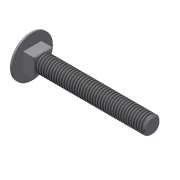
# Autodesk Inventor part: Šroub M10x70
Saved by Autodesk Inventor 2015 (Build 190159000, 159)
## iProperties
Created: 2015-07-31
Part Number: Šroub M10x70
Material: Všeobecné
Document SubType Name: Modeling
Designer: Michal
Density: 1 g/cm^3
Appearance: Výchozí
Author: Michal
Autodesk Inventor part; units mm, degrees
ref_plane "YZ Plane" through (0, 0, 0) normal (1, 0, 0) x (0, 1, 0)
ref_plane "XZ Plane" through (0, 0, 0) normal (0, 1, 0) x (-1, 0, 0)
ref_plane "XY Plane" through (0, 0, 0) normal (0, 0, 1) x (1, 0, 0)
sketch "Náčrt1" plane through (0, 0, 0) normal (0, 1, 0) x (-1, 0, 0)
  line L0 (0, 0) -> (0, 12)
  line L1 (0, 12) -> (1, 12)
  arc A0 (2.79, 0) -> (1, 12) centre (-37.5014, 0.1235) ccw
  line L2 (2.79, 0) -> (0, 0)
  dimension "d0" = 12
  dimension "d1" = 1
  constraints: 6 end point, 2 point on circle, 1 centre point, 1 horizontal, 1 perpendicular, 1 vertical
  measures "d0" distance of L0.start L0.end
  measures "d1" distance of L0.end L1.end
revolve "Rotace1" add sketch "Náčrt1" angle 360 about axis through (-2.79, 0, 0) along (1, 0, 0)
sketch "Náčrt2" plane through (0, 0, 0) normal (1, 0, 0) x (0, 0, -1)
  line L0 (-5.29, 5.29) -> (5.29, 5.29)
  line L1 (5.29, 5.29) -> (5.29, -5.29)
  line L2 (5.29, -5.29) -> (-5.29, -5.29)
  line L3 (-5.29, -5.29) -> (-5.29, 5.29)
  point P0 (0, 0)
  dimension "d3" = 10.58
  dimension "d4" = 10.58
  dimension "d5" = 5.29
  dimension "d6" = 5.29
  constraints: 8 end point, 2 parallel, 1 horizontal, 1 perpendicular
  measures "d3" distance of L1.end L2.end
  measures "d4" distance of L0.end L1.end
  measures "d5" distance from line of L1 point (0, 0)
  measures "d6" distance from line of L0 point (0, 0)
extrude "Vysunutí1" add sketch "Náčrt2" along normal blind 6.6
sketch "Náčrt3" plane through (6.6, 0, 0) normal (1, 0, 0) x (0, 0, -1)
  circle A0 centre (0, 0) radius 5
  dimension "d9" = 10
  constraints: 1 centre point, 1 coincident
  measures "d9" diameter of A0
extrude "Vysunutí2" add sketch "Náčrt3" along normal blind 63.4
chamfer "Zkosení1" distance 1 angle 45 1 edges at (70, 0, 5)
fillet "Zaoblení1" radius 1 4 edges at (6.6, 5.29, 0) (6.6, 0, 5.29) (6.6, -5.29, 0) (6.6, 0, -5.29)
thread "Závit1" size "M10x1.5" class "6g" standard "ANSI Metric M Profile" full length
